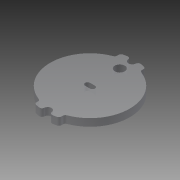
# Autodesk Inventor part: Outer Endcap080513
Saved by Autodesk Inventor 2013 SP1 (Build 170176100, 176)
## iProperties
Created: 2013-05-23
Part Number: Outer Endcap080513
Material: Polycarbonate, Clear
Document SubType Name: Modeling
Designer: Eric
Density: 1.2 g/cm^3
Mass: 2.90508 g
Surface Area: 20.2664 cm^2
Volume: 2.4209 cm^3
Author: Eric
Autodesk Inventor part; units mm, degrees
ref_plane "YZ Plane" through (0, 0, 0) normal (1, 0, 0) x (0, 1, 0)
ref_plane "XZ Plane" through (0, 0, 0) normal (0, 1, 0) x (-1, 0, 0)
ref_plane "XY Plane" through (0, 0, 0) normal (0, 0, 1) x (1, 0, 0)
sketch "Sketch1" plane through (0, 0, 0) normal (0, 0, 1) x (1, 0, 0)
  circle A0 centre (0, 12) radius 2
  arc A1 (-5.6471, 14.9703) -> (-5.6471, -14.9703) centre (0, 0) ccw
  arc A2 (5.6471, -14.9703) -> (5.6471, 14.9703) centre (0, 0) ccw
  line L0 (-5, -16.5227) -> (-5, -15.906)
  line L1 (-5, 15.906) -> (-5, 16.5227)
  line L2 (5, 16.5227) -> (5, 15.906)
  line L3 (5, -15.906) -> (5, -16.5227)
  arc A3 (-5.6471, 14.9703) -> (-5, 15.906) centre (-6, 15.906) ccw
  arc A4 (-4.2353, 17.4946) -> (-5, 16.5227) centre (-4, 16.5227) ccw
  arc A5 (5, 16.5227) -> (4.2353, 17.4946) centre (4, 16.5227) ccw
  arc A6 (5, 15.906) -> (5.6471, 14.9703) centre (6, 15.906) ccw
  arc A7 (5.6471, -14.9703) -> (5, -15.906) centre (6, -15.906) ccw
  arc A8 (4.2353, -17.4946) -> (5, -16.5227) centre (4, -16.5227) ccw
  arc A9 (-5, -16.5227) -> (-4.2353, -17.4946) centre (-4, -16.5227) ccw
  arc A10 (-5, -15.906) -> (-5.6471, -14.9703) centre (-6, -15.906) ccw
  arc A11 (-1.4959, 16.8897) -> (1.4959, 16.8897) centre (0, 17) ccw
  arc A12 (1.4959, -16.8897) -> (-1.4959, -16.8897) centre (0, -17) ccw
  arc A13 (4.2353, 17.4946) -> (2.6399, 17.8054) centre (0, 0) ccw
  arc A14 (-2.6399, 17.8054) -> (-4.2353, 17.4946) centre (0, 0) ccw
  arc A15 (-4.2353, -17.4946) -> (-2.6399, -17.8054) centre (0, 0) ccw
  arc A16 (2.6399, -17.8054) -> (4.2353, -17.4946) centre (0, 0) ccw
  arc A17 (-2.6399, -17.8054) -> (-1.4959, -16.8897) centre (-2.4932, -16.8162) ccw
  arc A18 (1.4959, -16.8897) -> (2.6399, -17.8054) centre (2.4932, -16.8162) ccw
  arc A19 (-1.4959, 16.8897) -> (-2.6399, 17.8054) centre (-2.4932, 16.8162) ccw
  arc A20 (2.6399, 17.8054) -> (1.4959, 16.8897) centre (2.4932, 16.8162) ccw
  arc A21 (-1, 1) -> (-1, -1) centre (-1, 0) ccw
  arc A22 (1, -1) -> (1, 1) centre (1, 0) ccw
  line L4 (-1, 1) -> (1, 1)
  line L5 (1, -1) -> (-1, -1)
  point P0 (-5, 17.2916)
  point P1 (5, -17.2916)
  point P2 (5, 17.2916)
  point P3 (-5, -17.2916)
  point P4 (5, 15.1987)
  point P5 (-5, 15.1987)
  point P6 (-5, -15.1987)
  point P7 (5, -15.1987)
  dimension "d6" = 4
  dimension "d16" = 1
  dimension "d17" = 16
  dimension "d18" = 16
  dimension "d21" = 10
  dimension "d22" = 10
  dimension "d25" = 3
  dimension "d28" = 3
  dimension "d29" = 1
  dimension "d34" = 12
  dimension "d35" = 2
  dimension "d36" = 2
  constraints: 48 point on circle, 23 centre point, 23 tangent, 12 end point, 10 equal radius, 8 point on line, 4 parallel, 1 coincident
  measures "d6" diameter of A0
  measures "d16" radius of A3
  measures "d17" radius of A1
  measures "d18" radius of A2
  measures "d21" distance between parallel lines of L1 L2
  measures "d22" distance between parallel lines of L3 L0
  measures "d25" diameter of A11
  measures "d28" diameter of A12
  measures "d29" radius of A17
  measures "d34" distance of point (0, 0) A0.centre
  measures "d35" diameter of A21
  measures "d36" diameter of A22
extrude "Extrusion4" add sketch "Sketch1" along normal blind 3
body "Solid4"
